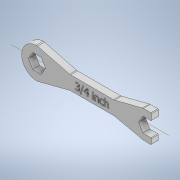
# Autodesk Inventor part: 3_4_inchWrenchV03
Saved by Autodesk Inventor 2020.2 (Build 242310000, 310)
## iProperties
Created: 2019-11-16
Part Number: 3_4_inchWrenchV03
Material: Generic
Document SubType Name: Modeling
Designer: steele
Density: 1 g/cm^3
Appearance: Default
Author: steele
Autodesk Inventor part; units mm, degrees
ref_plane "YZ Plane" through (0, 0, 0) normal (1, 0, 0) x (0, 1, 0)
ref_plane "XZ Plane" through (0, 0, 0) normal (0, 1, 0) x (-1, 0, 0)
ref_plane "XY Plane" through (0, 0, 0) normal (0, 0, 1) x (1, 0, 0)
sketch "Sketch2" plane through (0, 0, 0) normal (0, 0, 1) x (1, 0, 0)
  line L0 (-64.4682, 0) -> (-70.3341, -10.16)
  line L1 (-70.3341, -10.16) -> (-82.0659, -10.16)
  line L2 (-82.0659, -10.16) -> (-87.9318, 0)
  line L3 (-87.9318, 0) -> (-82.0659, 10.16)
  line L4 (-82.0659, 10.16) -> (-70.3341, 10.16)
  line L5 (-70.3341, 10.16) -> (-64.4682, 0)
  line L6 (-76.2, 0) -> (76.2, 0) construction
  line L7 (82.0659, -10.16) -> (70.3341, -10.16)
  line L8 (70.3341, -10.16) -> (64.4682, 0)
  line L9 (64.4682, 0) -> (70.3341, 10.16)
  line L10 (70.3341, 10.16) -> (82.0659, 10.16)
  line L11 (82.0659, 10.16) -> (82.4325, 9.525)
  line L12 (-132.627, 0) -> (135.7899, 0) projected
  line L13 (0, 0) -> (0, 37.2208) construction
  line L14 (0, 9.525) -> (30.4771, 9.525)
  line L15 (0, 9.525) -> (-30.4771, 9.525)
  circle A0 centre (-76.2, 0) radius 21.2568
  line L16 (-87.9318, 0) -> (-97.4568, 0) construction
  arc A1 (61.4802, 17.428) -> (59.9045, -15.9645) centre (76.2, 0) ccw
  line L17 (87.9318, 0) -> (97.4446, 0) construction
  line L18 (87.9318, 0) -> (89.9839, -16.166) construction
  line L19 (30.4771, 9.525) -> (70.3341, 19.685)
  line L20 (-76.2, 21.2568) -> (-30.4771, 9.525)
  line L21 (70.3341, 10.16) -> (70.3341, 19.685) construction
  line L22 (82.0659, 10.16) -> (82.0659, 19.685)
  line L23 (82.0659, -10.16) -> (81.717, -18.7112)
  line L24 (0, -9.525) -> (30.4771, -9.525)
  line L25 (0, -9.525) -> (-30.4771, -9.525)
  line L26 (30.4771, -9.525) -> (70.3341, -18.2468)
  line L27 (-76.2, -21.2568) -> (-30.4771, -9.525)
  line L28 (70.3341, 19.685) -> (82.0659, 19.685)
  line L29 (70.3341, -10.16) -> (70.3341, -18.2468) construction
  line L30 (70.3341, -18.2468) -> (81.717, -18.7112)
  point P0 (82.0659, 18.5801)
  point P1 (82.0659, -18.5801)
  dimension "centerToBoxEndWrench" = 76.2
  dimension "boltPrintedSize" = 20.32
  dimension "centerToOpenEndWrench" = 76.2
  dimension "d23" = 9.525
  dimension "d24" = 9.525
  dimension "d26" = 9.525
  constraints: 60 end point, 6 point on line, 5 horizontal, 5 symmetric about line, 4 point on circle, 4 vertical, 3 coincident, 3 collinear, 2 centre point, 2 perpendicular, 24 other
  measures "centerToBoxEndWrench" distance of L6.start L13.start
  measures "boltPrintedSize" distance between parallel lines of L1 L4
  measures "centerToOpenEndWrench" distance of L6.end L13.start
  measures "d23" distance between parallel lines of L14 L12
  measures "d24" distance of L16.end L2.end
  measures "d26" distance of L19.end L9.end
extrude "Extrusion2" add sketch "Sketch2" along normal mid plane 9.525 contours L12 A0 L27 L2 L1 L0 | L5 L4 L3 L12 A0 L20 | A0 L20 L15 L14 L19 A1 L12 | L12 A1 L26 L24 L25 L27 A0 | A1 L19 L28 L22 L10 L9 L12 | L12 L8 L7 L23 L30 L26 A1
fillet "Fillet1" radius 0.7937 4 edges at (82.0659, 19.685, 0) (82.0659, 10.16, 0) (82.0659, -10.16, 0) (81.717, -18.7112, 0)
fillet "Fillet2" radius 6.35 8 edges at (-30.4771, -9.525, 0) (30.4771, -9.525, 0) (70.3341, -18.2468, 0) (-76.2, -21.2568, 0) (-76.2, 21.2568, 0) (-30.4771, 9.525, 0) (30.4771, 9.525, 0) (70.3341, 19.685, 0)
sketch "Sketch3" plane through (0, 0, 4.7625) normal (0, 0, 1) x (1, 0, 0)
  line L0 (-64.4682, 0) -> (64.4682, 0) construction
  spline S0 degree 2 poles (-20.2541, 3.8594) (-20.6015, 3.8594) (-21.2885, 3.6896) (-21.6204, 3.5584) knots 0 0 0 1 2 2 2
  spline S1 degree 2 poles (-21.6204, 3.5584) (-21.9291, 3.4271) (-22.3845, 3.1493) (-22.5621, 3.0258) knots 0 0 0 1 2 2 2
  line L1 (-22.5621, 3.0258) -> (-22.6392, 3.0258)
  line L2 (-22.6392, 3.0258) -> (-22.6392, 4.3766)
  spline S2 degree 2 poles (-22.6392, 4.3766) (-22.2224, 4.6004) (-20.7944, 4.9632) (-20.1538, 4.9632) knots 0 0 0 1 2 2 2
  spline S3 degree 2 poles (-20.1538, 4.9632) (-19.5054, 4.9632) (-18.5406, 4.7007) (-18.1469, 4.4229) knots 0 0 0 1 2 2 2
  spline S4 degree 2 poles (-18.1469, 4.4229) (-17.7301, 4.1218) (-17.2978, 3.2496) (-17.2978, 2.663) knots 0 0 0 1 2 2 2
  spline S5 degree 2 poles (-17.2978, 2.663) (-17.2978, 1.8757) (-18.3322, 0.687) (-19.0577, 0.5326) knots 0 0 0 1 2 2 2
  line L3 (-19.0577, 0.5326) -> (-19.0577, 0.44)
  spline S6 degree 2 poles (-19.0577, 0.44) (-18.7567, 0.3782) (-18.0697, 0.1003) (-17.7764, -0.1775) knots 0 0 0 1 2 2 2
  spline S7 degree 2 poles (-17.7764, -0.1775) (-17.4831, -0.4477) (-17.1126, -1.3122) (-17.1126, -1.9374) knots 0 0 0 1 2 2 2
  spline S8 degree 2 poles (-17.1126, -1.9374) (-17.1126, -2.5781) (-17.5526, -3.6664) (-17.9539, -4.0832) knots 0 0 0 1 2 2 2
  spline S9 degree 2 poles (-17.9539, -4.0832) (-18.3707, -4.5155) (-19.5517, -4.9632) (-20.3004, -4.9632) knots 0 0 0 1 2 2 2
  spline S10 degree 2 poles (-20.3004, -4.9632) (-21.0183, -4.9632) (-22.4231, -4.6158) (-22.9017, -4.3766) knots 0 0 0 1 2 2 2
  line L4 (-22.9017, -4.3766) -> (-22.9017, -3.0258)
  line L5 (-22.9017, -3.0258) -> (-22.8091, -3.0258)
  spline S11 degree 2 poles (-22.8091, -3.0258) (-22.4077, -3.3191) (-21.0492, -3.8594) (-20.3776, -3.8594) knots 0 0 0 1 2 2 2
  spline S12 degree 2 poles (-20.3776, -3.8594) (-19.984, -3.8594) (-19.1967, -3.6124) (-18.9342, -3.3268) knots 0 0 0 1 2 2 2
  spline S13 degree 2 poles (-18.9342, -3.3268) (-18.6795, -3.0412) (-18.4093, -2.362) (-18.4093, -1.8448) knots 0 0 0 1 2 2 2
  spline S14 degree 2 poles (-18.4093, -1.8448) (-18.4093, -1.3276) (-18.7104, -0.6561) (-18.9805, -0.4631) knots 0 0 0 1 2 2 2
  spline S15 degree 2 poles (-18.9805, -0.4631) (-19.2507, -0.2702) (-19.984, -0.1235) (-20.4162, -0.1235) knots 0 0 0 1 2 2 2
  line L6 (-20.4162, -0.1235) -> (-20.9565, -0.1235)
  line L7 (-20.9565, -0.1235) -> (-20.9565, 0.934)
  line L8 (-20.9565, 0.934) -> (-20.532, 0.934)
  spline S16 degree 2 poles (-20.532, 0.934) (-19.6752, 0.934) (-18.5946, 1.7522) (-18.5946, 2.5318) knots 0 0 0 1 2 2 2
  spline S17 degree 2 poles (-18.5946, 2.5318) (-18.5946, 2.8946) (-18.8725, 3.4117) (-19.0963, 3.5661) knots 0 0 0 1 2 2 2
  spline S18 degree 2 poles (-19.0963, 3.5661) (-19.3356, 3.7282) (-19.9222, 3.8594) (-20.2541, 3.8594) knots 0 0 0 1 2 2 2
  line L9 (-11.7171, 5.187) -> (-15.4453, -6.8311)
  line L10 (-15.4453, -6.8311) -> (-16.526, -6.8311)
  line L11 (-16.526, -6.8311) -> (-12.8132, 5.187)
  line L12 (-12.8132, 5.187) -> (-11.7171, 5.187)
  line L13 (-4.5387, -1.4897) -> (-5.6733, -1.4897)
  line L14 (-5.6733, -1.4897) -> (-5.6733, -4.7625)
  line L15 (-5.6733, -4.7625) -> (-6.9006, -4.7625)
  line L16 (-6.9006, -4.7625) -> (-6.9006, -1.4897)
  line L17 (-6.9006, -1.4897) -> (-11.1074, -1.4897)
  line L18 (-11.1074, -1.4897) -> (-11.1074, -0.1467)
  line L19 (-11.1074, -0.1467) -> (-6.8466, 4.7625)
  line L20 (-6.8466, 4.7625) -> (-5.6733, 4.7625)
  line L21 (-5.6733, 4.7625) -> (-5.6733, -0.4631)
  line L22 (-5.6733, -0.4631) -> (-4.5387, -0.4631)
  line L23 (-4.5387, -0.4631) -> (-4.5387, -1.4897)
  line L24 (-6.9006, -0.4631) -> (-6.9006, 3.2573)
  line L25 (-6.9006, 3.2573) -> (-10.1039, -0.4631)
  line L26 (-10.1039, -0.4631) -> (-6.9006, -0.4631)
  line L27 (1.976, -4.7625) -> (0.7719, -4.7625)
  line L28 (0.7719, -4.7625) -> (0.7719, 2.3851)
  line L29 (0.7719, 2.3851) -> (1.976, 2.3851)
  line L30 (1.976, 2.3851) -> (1.976, -4.7625)
  line L31 (2.0609, 3.5738) -> (0.6947, 3.5738)
  line L32 (0.6947, 3.5738) -> (0.6947, 4.8243)
  line L33 (0.6947, 4.8243) -> (2.0609, 4.8243)
  line L34 (2.0609, 4.8243) -> (2.0609, 3.5738)
  line L35 (9.3552, -4.7625) -> (8.1511, -4.7625)
  line L36 (8.1511, -4.7625) -> (8.1511, -0.687)
  spline S19 degree 2 poles (8.1511, -0.687) (8.1511, -0.193) (8.0584, 0.6561) (7.9195, 0.9108) knots 0 0 0 1 2 2 2
  spline S20 degree 2 poles (7.9195, 0.9108) (7.7728, 1.181) (7.248, 1.4434) (6.8003, 1.4434) knots 0 0 0 1 2 2 2
  spline S21 degree 2 poles (6.8003, 1.4434) (6.3526, 1.4434) (5.4032, 0.9648) (4.9478, 0.5789) knots 0 0 0 1 2 2 2
  line L37 (4.9478, 0.5789) -> (4.9478, -4.7625)
  line L38 (4.9478, -4.7625) -> (3.7436, -4.7625)
  line L39 (3.7436, -4.7625) -> (3.7436, 2.3851)
  line L40 (3.7436, 2.3851) -> (4.9478, 2.3851)
  line L41 (4.9478, 2.3851) -> (4.9478, 1.5901)
  spline S22 degree 2 poles (4.9478, 1.5901) (5.4881, 2.0764) (6.5301, 2.5858) (7.1167, 2.5858) knots 0 0 0 1 2 2 2
  spline S23 degree 2 poles (7.1167, 2.5858) (8.1665, 2.5858) (9.3552, 1.1964) (9.3552, -0.1235) knots 0 0 0 1 2 2 2
  line L42 (9.3552, -0.1235) -> (9.3552, -4.7625)
  spline S24 degree 2 poles (13.8861, -4.9246) (13.1451, -4.9246) (11.9178, -4.4692) (11.4779, -4.0061) knots 0 0 0 1 2 2 2
  spline S25 degree 2 poles (11.4779, -4.0061) (11.0379, -3.5506) (10.5516, -2.1458) (10.5516, -1.2041) knots 0 0 0 1 2 2 2
  spline S26 degree 2 poles (10.5516, -1.2041) (10.5516, -0.2624) (11.0533, 1.1115) (11.4779, 1.5746) knots 0 0 0 1 2 2 2
  spline S27 degree 2 poles (11.4779, 1.5746) (11.9024, 2.0455) (13.1606, 2.5472) (13.8861, 2.5472) knots 0 0 0 1 2 2 2
  spline S28 degree 2 poles (13.8861, 2.5472) (14.4728, 2.5472) (15.5688, 2.2153) (15.9934, 1.9992) knots 0 0 0 1 2 2 2
  line L43 (15.9934, 1.9992) -> (15.9934, 0.6484)
  line L44 (15.9934, 0.6484) -> (15.9239, 0.6484)
  spline S29 degree 2 poles (15.9239, 0.6484) (15.7927, 0.7564) (15.3913, 1.0343) (15.1057, 1.181) knots 0 0 0 1 2 2 2
  spline S30 degree 2 poles (15.1057, 1.181) (14.851, 1.3045) (14.1717, 1.4974) (13.863, 1.4974) knots 0 0 0 1 2 2 2
  spline S31 degree 2 poles (13.863, 1.4974) (12.929, 1.4974) (11.7943, 0.0849) (11.7943, -1.2041) knots 0 0 0 1 2 2 2
  spline S32 degree 2 poles (11.7943, -1.2041) (11.7943, -2.4623) (12.8904, -3.8748) (13.863, -3.8748) knots 0 0 0 1 2 2 2
  spline S33 degree 2 poles (13.863, -3.8748) (14.4496, -3.8748) (15.5148, -3.3886) (15.9239, -3.0103) knots 0 0 0 1 2 2 2
  line L45 (15.9239, -3.0103) -> (15.9934, -3.0103)
  line L46 (15.9934, -3.0103) -> (15.9934, -4.3611)
  spline S34 degree 2 poles (15.9934, -4.3611) (15.8158, -4.446) (15.2755, -4.6853) (15.0594, -4.7393) knots 0 0 0 1 2 2 2
  spline S35 degree 2 poles (15.0594, -4.7393) (14.7506, -4.832) (14.2643, -4.9246) (13.8861, -4.9246) knots 0 0 0 1 2 2 2
  line L47 (22.701, -4.7625) -> (21.4969, -4.7625)
  line L48 (21.4969, -4.7625) -> (21.4969, -0.687)
  spline S36 degree 2 poles (21.4969, -0.687) (21.4969, -0.193) (21.4042, 0.6561) (21.2653, 0.9108) knots 0 0 0 1 2 2 2
  spline S37 degree 2 poles (21.2653, 0.9108) (21.1186, 1.181) (20.5938, 1.4434) (20.1461, 1.4434) knots 0 0 0 1 2 2 2
  spline S38 degree 2 poles (20.1461, 1.4434) (19.6984, 1.4434) (18.749, 0.9648) (18.2936, 0.5789) knots 0 0 0 1 2 2 2
  line L49 (18.2936, 0.5789) -> (18.2936, -4.7625)
  line L50 (18.2936, -4.7625) -> (17.0894, -4.7625)
  line L51 (17.0894, -4.7625) -> (17.0894, 5.187)
  line L52 (17.0894, 5.187) -> (18.2936, 5.187)
  line L53 (18.2936, 5.187) -> (18.2936, 1.5901)
  spline S39 degree 2 poles (18.2936, 1.5901) (18.8339, 2.0764) (19.8759, 2.5858) (20.4625, 2.5858) knots 0 0 0 1 2 2 2
  spline S40 degree 2 poles (20.4625, 2.5858) (21.5123, 2.5858) (22.701, 1.1964) (22.701, -0.1235) knots 0 0 0 1 2 2 2
  line L54 (22.701, -0.1235) -> (22.701, -4.7625)
  point P0 (0, 0)
  constraints: 2 end point, 2 horizontal
extrude "Extrusion3" cut sketch "Sketch3" against normal blind 3.175
sketch "Sketch6" plane through (0, 0, -4.7625) normal (0, 0, -1) x (-1, 0, 0)
  line L0 (-64.4682, 0) -> (65.0757, 0) construction
  spline S0 degree 2 poles (-19.9504, 3.8594) (-20.2977, 3.8594) (-20.9847, 3.6896) (-21.3166, 3.5584) knots 0 0 0 1 2 2 2
  spline S1 degree 2 poles (-21.3166, 3.5584) (-21.6254, 3.4271) (-22.0808, 3.1493) (-22.2583, 3.0258) knots 0 0 0 1 2 2 2
  line L1 (-22.2583, 3.0258) -> (-22.3355, 3.0258)
  line L2 (-22.3355, 3.0258) -> (-22.3355, 4.3766)
  spline S2 degree 2 poles (-22.3355, 4.3766) (-21.9187, 4.6004) (-20.4907, 4.9632) (-19.8501, 4.9632) knots 0 0 0 1 2 2 2
  spline S3 degree 2 poles (-19.8501, 4.9632) (-19.2017, 4.9632) (-18.2368, 4.7007) (-17.8432, 4.4229) knots 0 0 0 1 2 2 2
  spline S4 degree 2 poles (-17.8432, 4.4229) (-17.4263, 4.1218) (-16.9941, 3.2496) (-16.9941, 2.663) knots 0 0 0 1 2 2 2
  spline S5 degree 2 poles (-16.9941, 2.663) (-16.9941, 1.8757) (-18.0284, 0.687) (-18.754, 0.5326) knots 0 0 0 1 2 2 2
  line L3 (-18.754, 0.5326) -> (-18.754, 0.44)
  spline S6 degree 2 poles (-18.754, 0.44) (-18.4529, 0.3782) (-17.766, 0.1003) (-17.4727, -0.1775) knots 0 0 0 1 2 2 2
  spline S7 degree 2 poles (-17.4727, -0.1775) (-17.1793, -0.4477) (-16.8088, -1.3122) (-16.8088, -1.9374) knots 0 0 0 1 2 2 2
  spline S8 degree 2 poles (-16.8088, -1.9374) (-16.8088, -2.5781) (-17.2488, -3.6664) (-17.6502, -4.0832) knots 0 0 0 1 2 2 2
  spline S9 degree 2 poles (-17.6502, -4.0832) (-18.067, -4.5155) (-19.248, -4.9632) (-19.9967, -4.9632) knots 0 0 0 1 2 2 2
  spline S10 degree 2 poles (-19.9967, -4.9632) (-20.7146, -4.9632) (-22.1194, -4.6158) (-22.5979, -4.3766) knots 0 0 0 1 2 2 2
  line L4 (-22.5979, -4.3766) -> (-22.5979, -3.0258)
  line L5 (-22.5979, -3.0258) -> (-22.5053, -3.0258)
  spline S11 degree 2 poles (-22.5053, -3.0258) (-22.1039, -3.3191) (-20.7454, -3.8594) (-20.0739, -3.8594) knots 0 0 0 1 2 2 2
  spline S12 degree 2 poles (-20.0739, -3.8594) (-19.6802, -3.8594) (-18.8929, -3.6124) (-18.6305, -3.3268) knots 0 0 0 1 2 2 2
  spline S13 degree 2 poles (-18.6305, -3.3268) (-18.3758, -3.0412) (-18.1056, -2.362) (-18.1056, -1.8448) knots 0 0 0 1 2 2 2
  spline S14 degree 2 poles (-18.1056, -1.8448) (-18.1056, -1.3276) (-18.4066, -0.6561) (-18.6768, -0.4631) knots 0 0 0 1 2 2 2
  spline S15 degree 2 poles (-18.6768, -0.4631) (-18.947, -0.2702) (-19.6802, -0.1235) (-20.1125, -0.1235) knots 0 0 0 1 2 2 2
  line L6 (-20.1125, -0.1235) -> (-20.6528, -0.1235)
  line L7 (-20.6528, -0.1235) -> (-20.6528, 0.934)
  line L8 (-20.6528, 0.934) -> (-20.2283, 0.934)
  spline S16 degree 2 poles (-20.2283, 0.934) (-19.3715, 0.934) (-18.2909, 1.7522) (-18.2909, 2.5318) knots 0 0 0 1 2 2 2
  spline S17 degree 2 poles (-18.2909, 2.5318) (-18.2909, 2.8946) (-18.5687, 3.4117) (-18.7926, 3.5661) knots 0 0 0 1 2 2 2
  spline S18 degree 2 poles (-18.7926, 3.5661) (-19.0319, 3.7282) (-19.6185, 3.8594) (-19.9504, 3.8594) knots 0 0 0 1 2 2 2
  line L9 (-11.4134, 5.187) -> (-15.1416, -6.8311)
  line L10 (-15.1416, -6.8311) -> (-16.2222, -6.8311)
  line L11 (-16.2222, -6.8311) -> (-12.5095, 5.187)
  line L12 (-12.5095, 5.187) -> (-11.4134, 5.187)
  line L13 (-4.2349, -1.4897) -> (-5.3696, -1.4897)
  line L14 (-5.3696, -1.4897) -> (-5.3696, -4.7625)
  line L15 (-5.3696, -4.7625) -> (-6.5969, -4.7625)
  line L16 (-6.5969, -4.7625) -> (-6.5969, -1.4897)
  line L17 (-6.5969, -1.4897) -> (-10.8036, -1.4897)
  line L18 (-10.8036, -1.4897) -> (-10.8036, -0.1467)
  line L19 (-10.8036, -0.1467) -> (-6.5428, 4.7625)
  line L20 (-6.5428, 4.7625) -> (-5.3696, 4.7625)
  line L21 (-5.3696, 4.7625) -> (-5.3696, -0.4631)
  line L22 (-5.3696, -0.4631) -> (-4.2349, -0.4631)
  line L23 (-4.2349, -0.4631) -> (-4.2349, -1.4897)
  line L24 (-6.5969, -0.4631) -> (-6.5969, 3.2573)
  line L25 (-6.5969, 3.2573) -> (-9.8002, -0.4631)
  line L26 (-9.8002, -0.4631) -> (-6.5969, -0.4631)
  line L27 (2.2797, -4.7625) -> (1.0756, -4.7625)
  line L28 (1.0756, -4.7625) -> (1.0756, 2.3851)
  line L29 (1.0756, 2.3851) -> (2.2797, 2.3851)
  line L30 (2.2797, 2.3851) -> (2.2797, -4.7625)
  line L31 (2.3647, 3.5738) -> (0.9984, 3.5738)
  line L32 (0.9984, 3.5738) -> (0.9984, 4.8243)
  line L33 (0.9984, 4.8243) -> (2.3647, 4.8243)
  line L34 (2.3647, 4.8243) -> (2.3647, 3.5738)
  line L35 (9.6589, -4.7625) -> (8.4548, -4.7625)
  line L36 (8.4548, -4.7625) -> (8.4548, -0.687)
  spline S19 degree 2 poles (8.4548, -0.687) (8.4548, -0.193) (8.3622, 0.6561) (8.2232, 0.9108) knots 0 0 0 1 2 2 2
  spline S20 degree 2 poles (8.2232, 0.9108) (8.0766, 1.181) (7.5517, 1.4434) (7.104, 1.4434) knots 0 0 0 1 2 2 2
  spline S21 degree 2 poles (7.104, 1.4434) (6.6563, 1.4434) (5.7069, 0.9648) (5.2515, 0.5789) knots 0 0 0 1 2 2 2
  line L37 (5.2515, 0.5789) -> (5.2515, -4.7625)
  line L38 (5.2515, -4.7625) -> (4.0474, -4.7625)
  line L39 (4.0474, -4.7625) -> (4.0474, 2.3851)
  line L40 (4.0474, 2.3851) -> (5.2515, 2.3851)
  line L41 (5.2515, 2.3851) -> (5.2515, 1.5901)
  spline S22 degree 2 poles (5.2515, 1.5901) (5.7918, 2.0764) (6.8338, 2.5858) (7.4205, 2.5858) knots 0 0 0 1 2 2 2
  spline S23 degree 2 poles (7.4205, 2.5858) (8.4702, 2.5858) (9.6589, 1.1964) (9.6589, -0.1235) knots 0 0 0 1 2 2 2
  line L42 (9.6589, -0.1235) -> (9.6589, -4.7625)
  spline S24 degree 2 poles (14.1899, -4.9246) (13.4489, -4.9246) (12.2216, -4.4692) (11.7816, -4.0061) knots 0 0 0 1 2 2 2
  spline S25 degree 2 poles (11.7816, -4.0061) (11.3416, -3.5506) (10.8553, -2.1458) (10.8553, -1.2041) knots 0 0 0 1 2 2 2
  spline S26 degree 2 poles (10.8553, -1.2041) (10.8553, -0.2624) (11.3571, 1.1115) (11.7816, 1.5746) knots 0 0 0 1 2 2 2
  spline S27 degree 2 poles (11.7816, 1.5746) (12.2061, 2.0455) (13.4643, 2.5472) (14.1899, 2.5472) knots 0 0 0 1 2 2 2
  spline S28 degree 2 poles (14.1899, 2.5472) (14.7765, 2.5472) (15.8726, 2.2153) (16.2971, 1.9992) knots 0 0 0 1 2 2 2
  line L43 (16.2971, 1.9992) -> (16.2971, 0.6484)
  line L44 (16.2971, 0.6484) -> (16.2276, 0.6484)
  spline S29 degree 2 poles (16.2276, 0.6484) (16.0964, 0.7564) (15.695, 1.0343) (15.4094, 1.181) knots 0 0 0 1 2 2 2
  spline S30 degree 2 poles (15.4094, 1.181) (15.1547, 1.3045) (14.4755, 1.4974) (14.1667, 1.4974) knots 0 0 0 1 2 2 2
  spline S31 degree 2 poles (14.1667, 1.4974) (13.2327, 1.4974) (12.0981, 0.0849) (12.0981, -1.2041) knots 0 0 0 1 2 2 2
  spline S32 degree 2 poles (12.0981, -1.2041) (12.0981, -2.4623) (13.1941, -3.8748) (14.1667, -3.8748) knots 0 0 0 1 2 2 2
  spline S33 degree 2 poles (14.1667, -3.8748) (14.7533, -3.8748) (15.8185, -3.3886) (16.2276, -3.0103) knots 0 0 0 1 2 2 2
  line L45 (16.2276, -3.0103) -> (16.2971, -3.0103)
  line L46 (16.2971, -3.0103) -> (16.2971, -4.3611)
  spline S34 degree 2 poles (16.2971, -4.3611) (16.1196, -4.446) (15.5792, -4.6853) (15.3631, -4.7393) knots 0 0 0 1 2 2 2
  spline S35 degree 2 poles (15.3631, -4.7393) (15.0544, -4.832) (14.5681, -4.9246) (14.1899, -4.9246) knots 0 0 0 1 2 2 2
  line L47 (23.0047, -4.7625) -> (21.8006, -4.7625)
  line L48 (21.8006, -4.7625) -> (21.8006, -0.687)
  spline S36 degree 2 poles (21.8006, -0.687) (21.8006, -0.193) (21.708, 0.6561) (21.569, 0.9108) knots 0 0 0 1 2 2 2
  spline S37 degree 2 poles (21.569, 0.9108) (21.4224, 1.181) (20.8975, 1.4434) (20.4498, 1.4434) knots 0 0 0 1 2 2 2
  spline S38 degree 2 poles (20.4498, 1.4434) (20.0021, 1.4434) (19.0527, 0.9648) (18.5973, 0.5789) knots 0 0 0 1 2 2 2
  line L49 (18.5973, 0.5789) -> (18.5973, -4.7625)
  line L50 (18.5973, -4.7625) -> (17.3932, -4.7625)
  line L51 (17.3932, -4.7625) -> (17.3932, 5.187)
  line L52 (17.3932, 5.187) -> (18.5973, 5.187)
  line L53 (18.5973, 5.187) -> (18.5973, 1.5901)
  spline S39 degree 2 poles (18.5973, 1.5901) (19.1376, 2.0764) (20.1796, 2.5858) (20.7663, 2.5858) knots 0 0 0 1 2 2 2
  spline S40 degree 2 poles (20.7663, 2.5858) (21.816, 2.5858) (23.0047, 1.1964) (23.0047, -0.1235) knots 0 0 0 1 2 2 2
  line L54 (23.0047, -0.1235) -> (23.0047, -4.7625)
  point P0 (0, 0)
  constraints: 2 end point, 2 horizontal
extrude "Extrusion4" cut sketch "Sketch6" against normal blind 3.175
equation "\"centerToBoxEndWrench\" = 4 * boltSize"
equation "\"boltPrintedSize\" = boltSize + boltGap"
equation "\"centerToOpenEndWrench\" = 4 * boltSize"
equation "\"d23\" = 0.5 * boltSize"
equation "\"d24\" = minWallThickness"
equation "\"d26\" = minWallThickness"
equation "\"d27\" = minWallThickness"
equation "\"textDepth\" = 0.333333 * minWallThickness"
equation "\"d33\" = textDepth"
equation "\"minWallThickness\" = 9.525"
equation "\"boltGap\" = 1.27"
equation "\"boltSize\" = 19.05"
body "Solid2"
